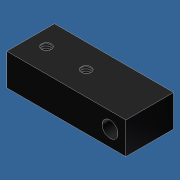
# Autodesk Inventor part: GE-12023
Saved by Autodesk Inventor 2012 (Build 160160000, 160)
## iProperties
Created: 2011-06-15
Part Number: GE-12023
Document SubType Name: Modeling
Designer: dfoster
Density: 1 g/cm^3
Description: Hinge Plate, Single
Mass: 84.9248 g
Surface Area: 163.524 cm^2
Volume: 84.9248 cm^3
Material: Default
Title: Hinge Plate, Single
Author: dfoster
Autodesk Inventor part; units mm, degrees
ref_plane "YZ Plane" through (0, 0, 0) normal (1, 0, 0) x (0, 1, 0)
ref_plane "XZ Plane" through (0, 0, 0) normal (0, 1, 0) x (-1, 0, 0)
ref_plane "XY Plane" through (0, 0, 0) normal (0, 0, 1) x (1, 0, 0)
sketch "Sketch1" plane through (0, 0, 0) normal (0, 0, 1) x (1, 0, 0)
  line L0 (0, 0) -> (95.25, 0)
  line L1 (95.25, 0) -> (95.25, 25.4)
  line L2 (95.25, 25.4) -> (0, 25.4)
  line L3 (0, 25.4) -> (0, 0)
  circle A0 centre (82.55, 12.7) radius 6.35
  dimension "d0" = 25.4
  dimension "d1" = 95.25
  dimension "d2" = 12.7
  dimension "d3" = 12.7
  dimension "d4" = 12.7
  constraints: 8 end point, 2 parallel, 1 centre point, 1 horizontal, 1 perpendicular
  measures "d0" distance between parallel lines of L0 L2
  measures "d1" distance of L1.end L2.end
  measures "d2" diameter of A0
  measures "d3" distance from line of A0.centre L2
  measures "d4" distance from line of A0.centre L1
extrude "Extrusion1" add sketch "Sketch1" along normal blind 38.1
hole "Hole1" at (12.7, 25.4, 19.05) direction (0, -1, 0) diameter 7.7978 end through all thread size "3/8-16 UNC" class "2B" standard "ANSI Unified Screw Threads"
pattern_linear "Rectangular Pattern1" count 2 spacing 31.75 along (1, 0, 0) of "Hole1"
equation "\"d3\" = 0.5 * d0"
equation "\"d4\" = d3"
body "Solid1"
